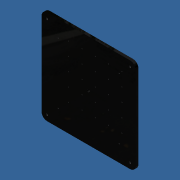
# Autodesk Inventor part: J007127
Saved by Autodesk Inventor 2018.2 (Build 222227000, 227)
## iProperties
Created: 2014-04-04
Material: ALUMINUM, 6061-T651
Vendor: HHMI: JFRC - ID&F
Document SubType Name: Modeling
Designer: NEGRASHOVI
Density: 2.7 g/cm^3
Mass: 791.664 g
Surface Area: 995.923 cm^2
Volume: 293.209 cm^3
Description: RGB PCB SUPPORT
Appearance: Glossy - Black
Part Number: J007127
Project: P-298001
RuleStatus: InUse
AfterDocSave0: file://Part Number Cleaner
LAB/DEPT: RUBIN (LAB)
REQUESTING SCIENTIST: ASO, YOSHI
SURFACE ROUGHNESS: 32 ra
DESIGN DEPARTMENT: HHMI: JRC - ID&F
SPECIAL FINISH: ANODIZE PER MIL-A-8625F, TYPE II, CLASS 2 (BLACK)
ALTERED ITEM PART NUMBER: N/A
ALTERED ITEM VENDOR: N/A
ALTERED ITEM DESCRIPTION: N/A
Author: NEGRASHOVI
Revision Number: -
Autodesk Inventor part; units mm, degrees
ref_plane "YZ Plane" through (0, 0, 0) normal (1, 0, 0) x (0, 1, 0)
ref_plane "XZ Plane" through (0, 0, 0) normal (0, 1, 0) x (-1, 0, 0)
ref_plane "XY Plane" through (0, 0, 0) normal (0, 0, 1) x (1, 0, 0)
sketch "Sketch1" plane through (0, 0, 0) normal (0, 0, 1) x (1, 0, 0)
  line L0 (-95.25, -107.95) -> (95.25, -107.95)
  line L1 (107.95, -95.25) -> (107.95, 95.25)
  line L2 (95.25, 107.95) -> (-95.25, 107.95)
  line L3 (-107.95, 95.25) -> (-107.95, -95.25)
  arc A0 (-95.25, 107.95) -> (-107.95, 95.25) centre (-95.25, 95.25) ccw
  arc A1 (107.95, 95.25) -> (95.25, 107.95) centre (95.25, 95.25) ccw
  arc A2 (95.25, -107.95) -> (107.95, -95.25) centre (95.25, -95.25) ccw
  arc A3 (-107.95, -95.25) -> (-95.25, -107.95) centre (-95.25, -95.25) ccw
  line L4 (-69.85, 69.85) -> (69.85, 69.85) construction
  line L5 (69.85, 69.85) -> (69.85, -69.85) construction
  line L6 (69.85, -69.85) -> (-69.85, -69.85) construction
  line L7 (-69.85, -69.85) -> (-69.85, 69.85) construction
  line L8 (-154.8124, 0) -> (154.8124, 0) construction
  line L9 (0, -154.8124) -> (0, 154.8124) construction
  point P0 (0, 0)
  point P1 (-107.95, -107.95)
  point P2 (107.95, 107.95)
  point P3 (107.95, -107.95)
  point P4 (-107.95, 107.95)
  point P5 (0, 0)
  point P6 (0, 107.95)
  point P7 (107.95, 0)
  point P8 (0, 0)
  point P9 (69.85, 0)
  point P10 (0, 69.85)
  point P11 (-45.72, -45.72)
  point P12 (-45.72, -15.24)
  point P13 (-45.72, 15.24)
  point P14 (-45.72, 45.72)
  point P15 (-45.72, 76.2)
  point P16 (-15.24, -45.72)
  point P17 (-15.24, -15.24)
  point P18 (-15.24, 15.24)
  point P19 (-15.24, 45.72)
  point P20 (-15.24, 76.2)
  point P21 (15.24, -45.72)
  point P22 (15.24, -15.24)
  point P23 (15.24, 15.24)
  point P24 (15.24, 45.72)
  point P25 (15.24, 76.2)
  point P26 (45.72, -45.72)
  point P27 (45.72, -15.24)
  point P28 (45.72, 15.24)
  point P29 (45.72, 45.72)
  point P30 (45.72, 76.2)
  point P31 (76.2, -45.72)
  point P32 (76.2, -15.24)
  point P33 (76.2, 15.24)
  point P34 (76.2, 45.72)
  point P35 (76.2, 76.2)
  dimension "d0" = 215.9
  dimension "d1" = 215.9
  dimension "d46" = 12.7
  dimension "d61" = 139.7
  dimension "d62" = 139.7
  dimension "d65" = 30.48
  dimension "d68" = 30.48
  constraints: 16 end point, 10 coincident, 8 point on circle, 8 point on line, 8 tangent, 4 centre point, 4 midpoint, 4 parallel, 3 equal radius, 3 horizontal, 2 horizontal alignment, 2 perpendicular, 2 symmetric about line, 2 vertical alignment, 1 vertical, 24 other
  measures "d0" distance of point (107.95, 107.95) point (-107.95, 107.95)
  measures "d1" distance of point (107.95, -107.95) point (107.95, 107.95)
  measures "d46" radius of A0
  measures "d61" distance of L4.start L4.end
  measures "d62" distance of L4.end L5.end
  measures "d65" distance of point (-45.72, -45.72) point (-45.72, -15.24)
  measures "d68" distance of point (-45.72, -45.72) point (-15.24, -45.72)
extrude "Extrusion1" add sketch "Sketch1" along normal blind 6.35
hole "Hole5" at (-95.25, 95.25, 0) at (95.25, 95.25, 0) at (95.25, -95.25, 0) at (-95.25, -95.25, 0) direction (0, 0, 1) diameter 4.9784 end through all thread size "1/4-20 UNC" class "2B" standard "ANSI Unified Screw Threads"
hole "Hole6" at (0, 0, 0) direction (0, 0, 1) diameter 6.7996 end through all
hole "Hole7" at (-45.72, -45.72, 0) at (-45.72, -15.24, 0) at (-45.72, 15.24, 0) at (-45.72, 45.72, 0) at (-45.72, 76.2, 0) at (-15.24, -45.72, 0) at (-15.24, -15.24, 0) at (-15.24, 15.24, 0) at (-15.24, 45.72, 0) at (-15.24, 76.2, 0) at (15.24, -45.72, 0) at (15.24, -15.24, 0) at (15.24, 15.24, 0) at (15.24, 45.72, 0) at (15.24, 76.2, 0) at (45.72, -45.72, 0) at (45.72, -15.24, 0) at (45.72, 15.24, 0) at (45.72, 45.72, 0) at (45.72, 76.2, 0) at (76.2, -45.72, 0) at (76.2, -15.24, 0) at (76.2, 15.24, 0) at (76.2, 45.72, 0) at (76.2, 76.2, 0) direction (0, 0, 1) diameter 2.159 end through all
hole "Hole8" at (69.85, 69.85, 0) at (-69.85, 69.85, 0) at (-69.85, -69.85, 0) at (69.85, -69.85, 0) direction (0, 0, 1) diameter 2.6416 end through all thread size "6-32 UNC" class "2B" standard "ANSI Unified Screw Threads"
equation "\"d1\" = d0"
equation "\"d62\" = d61"
body "Solid1"
